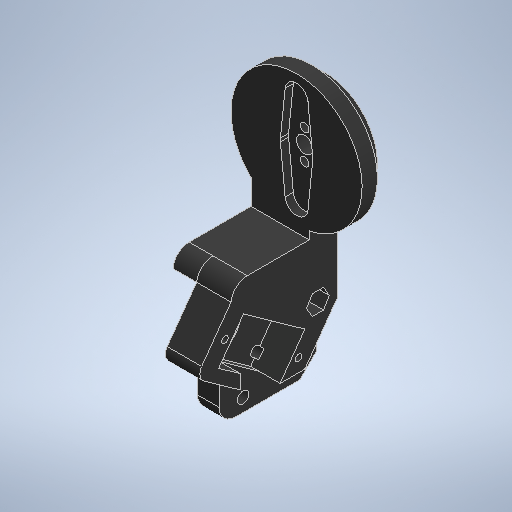
# Autodesk Inventor part: BracoRobotico_0008_001
Saved by Autodesk Inventor 2025.2 (Build 292293000, 293)
## iProperties
Created: 2025-05-22
Part Number: BracoRobotico_0008_001
Material: Rubber
Document SubType Name: Modeling
Designer: I
Density: 0.93 g/cm^3
Appearance: Rubber - Black
Author: I
Autodesk Inventor part; units mm, degrees
sketch "Sketch45" plane through (0, 0, 0) normal (0, 0, 1) x (1, 0, 0)
  circle A0 centre (0, 0) radius 20
  dimension "d321" = 40
  constraints: 1 centre point, 1 coincident
  measures "d321" diameter of A0
extrude "Extrusion48" add sketch "Sketch45" along normal mid plane 8.65
sketch "Sketch49" plane through (0, 0, 4.325) normal (0, 0, 1) x (1, 0, 0)
  circle A0 centre (0, 0) radius 2.5
  circle A1 centre (0, -4.5) radius 1.3
  circle A2 centre (0, 4.5) radius 1.3
  line L0 (0, -4.5) -> (0, 4.5) construction
  circle A3 centre (0, -14) radius 3.5 construction
  circle A4 centre (0, 14) radius 3.5 construction
  line L1 (0, -14) -> (0, 14) construction
  circle A5 centre (0, 0) radius 4.95 construction
  line L2 (-3.4812, -14.3625) -> (-4.9234, -0.5127)
  line L3 (3.4812, -14.3625) -> (4.9234, -0.5127)
  line L4 (-4.9234, 0.5127) -> (-3.4812, 14.3625)
  line L5 (4.9234, 0.5127) -> (3.4812, 14.3625)
  arc A6 (-3.4812, -14.3625) -> (3.4812, -14.3625) centre (0, -14) ccw
  arc A7 (3.4812, 14.3625) -> (-3.4812, 14.3625) centre (0, 14) ccw
  arc A8 (-4.9234, 0.5127) -> (-4.9234, -0.5127) centre (0, 0) ccw
  arc A9 (4.9234, -0.5127) -> (4.9234, 0.5127) centre (0, 0) ccw
  dimension "d338" = 5
  dimension "d339" = 9
  dimension "d340" = 2.6
  dimension "d343" = 7
  dimension "d344" = 28
  dimension "d345" = 9.9
  constraints: 16 point on circle, 12 end point, 10 centre point, 8 tangent, 7 coincident, 2 equal radius, 2 midpoint, 2 vertical
  measures "d338" diameter of A0
  measures "d339" distance of L0.start L0.end
  measures "d340" diameter of A1
  measures "d343" diameter of A4
  measures "d344" distance of L1.start L1.end
  measures "d345" diameter of A5
extrude "Extrusion52" cut sketch "Sketch49" along normal through all both and the other way through all contours A0 | A1 | A2
extrude "Extrusion53" cut sketch "Sketch49" against normal blind 2.5
sketch "Sketch50" plane through (0, 0, -4.325) normal (0, 0, -1) x (-1, 0, 0)
  circle A0 centre (0, -4.5) radius 1.3 construction
  circle A1 centre (0, 4.5) radius 1.3 construction
  circle A2 centre (0, 4.5) radius 3
  circle A3 centre (0, -4.5) radius 3
  point P0 (0, 0)
  dimension "d348" = 6
  constraints: 2 centre point, 2 coincident, 1 equal radius
  measures "d348" diameter of A2
extrude "Extrusion54" cut sketch "Sketch50" against normal blind 3
sketch "Sketch52" plane through (0, 0, -4.325) normal (0, 0, -1) x (-1, 0, 0)
  line L0 (-3.875, -22) -> (13.875, -22)
  line L1 (13.875, -22) -> (13.875, -64)
  line L2 (13.875, -64) -> (-3.875, -64)
  line L3 (-3.875, -64) -> (-3.875, -22)
  line L4 (-3.875, -22) -> (13.875, -64) construction
  line L5 (13.875, -22) -> (-3.875, -64) construction
  point P0 (0, 0)
  point P1 (5, -43)
  dimension "d354" = 17.75
  dimension "d355" = 5
  dimension "d357" = 64
  dimension "d358" = 22
  constraints: 12 end point, 2 midpoint, 1 perpendicular, 1 vertical
  measures "d354" distance of L1.end L2.end
  measures "d355" horizontal distance of point (5, -43) point (0, 0)
  measures "d357" distance from line of point (0, 0) L2
  measures "d358" distance from line of point (0, 0) L0
extrude "Extrusion55" add sketch "Sketch52" against normal blind 40.5
sketch "Sketch54" plane through (0, 0, -4.325) normal (0, 0, -1) x (-1, 0, 0)
  line L0 (13.875, -22) -> (-3.875, -22) projected
  circle A0 centre (0, 0) radius 20 projected
  line L1 (13.875, -22) -> (13.875, -14.4043)
  line L2 (-3.875, -22) -> (-3.875, -19.621)
  constraints: 4 end point, 2 point on circle, 2 vertical
extrude "Extrusion56" add sketch "Sketch54" against normal up to surface (8.65 mm away) contours L0 L2 A0 L1
sketch "Sketch55" plane through (-13.875, -64, -4.325) normal (-1, 0, 0) x (0, 0, 1)
  circle A0 centre (16, 36.748) radius 1.5
  circle A1 centre (16, 11.7287) radius 1.5
  line L0 (0, 0) -> (0, 49.5957) construction
  line L1 (0, 37.5) -> (0, 14.5)
  circle A2 centre (6, 24.2978) radius 1.5
  arc A3 (14.6844, 34.2416) -> (6, 37.5) centre (6, 24.2978) ccw
  line L2 (6, 37.5) -> (0, 37.5)
  line L3 (0, 14.5) -> (1.0053, 13.3867)
  arc A4 (1.0053, 13.3867) -> (14.8889, 16.2363) centre (6, 24.2978) ccw
  arc A5 (17.1111, 16.2363) -> (14.8889, 16.2363) centre (16, 15.2287) ccw
  arc A6 (14.6844, 34.2416) -> (17.3156, 34.2416) centre (16, 35.748) ccw
  circle A7 centre (26, 24.2978) radius 12 construction
  arc A8 (17.1111, 16.2363) -> (29.6085, 12.8532) centre (26, 24.2978) ccw
  arc A9 (26, 37.5) -> (17.3156, 34.2416) centre (26, 24.2978) ccw
  line L4 (26, 37.5) -> (40.5, 37.5)
  line L5 (40.5, 42) -> (40.5, 0) construction
  line L6 (26, 24.2978) -> (29.6085, 12.8532) construction
  line L7 (26, 24.2978) -> (26, 37.5) construction
  line L8 (29.6085, 12.8532) -> (40.5, 12.8532)
  line L9 (40.5, 37.5) -> (40.5, 12.8532)
  point P0 (4.325, 64)
  point P1 (0, 26)
  point P2 (0, 24.7978)
  dimension "d363" = 3
  dimension "d369" = 23
  dimension "d370" = 3
  dimension "d371" = 6
  dimension "d372" = 0.5
  dimension "d375" = 38
  dimension "d377" = 12
  dimension "d378" = 1.5
  dimension "d383" = 1.5
  dimension "d384" = 3.5
  dimension "d385" = 1
  dimension "d386" = 2
  dimension "d388" = 24
  dimension "d389" = 162.5
  dimension "d392" = 20
  constraints: 16 end point, 14 point on circle, 10 centre point, 5 vertical alignment, 4 coincident, 4 point on line, 4 tangent, 3 horizontal, 2 horizontal alignment, 2 midpoint, 1 equal radius
  measures "d363" diameter of A0
  measures "d369" distance of L1.start L1.end
  measures "d370" diameter of A2
  measures "d371" distance from line of L0 A2.centre
  measures "d372" vertical distance of point (0, 24.798) A2.centre
  measures "d375" vertical distance of point (4.325, 64) point (0, 26)
  measures "d377" radius of A4
  measures "d378" distance of L1.end L3.end
  measures "d383" radius of A5
  measures "d384" distance of A1.centre A5.centre
  measures "d385" distance of A0.centre A6.centre
  measures "d386" radius of A6
  measures "d388" diameter of A7
  measures "d389" angle of L7 L6
  measures "d392" distance of A2.centre A7.centre
extrude "Extrusion57" cut sketch "Sketch55" against normal blind 10 contours A0 | A1
extrude "Extrusion58" cut sketch "Sketch55" against normal blind 7.25 contours L2 A3 A6 A9 L4 L9 L8 A8 A5 A4 L3 L1 | A2
extrude "Extrusion59" cut sketch "Sketch55" along normal through all both and the other way through all contours A2
sketch "Sketch56" plane through (-6.625, -22, 4.325) normal (-1, 0, 0) x (0, 0, 1)
  line L0 (32.8095, -17.0077) -> (23.85, -4.5)
  line L1 (23.85, -4.5) -> (23.85, 0)
  line L2 (0, 0) -> (31.85, 0) construction
  line L3 (-8.65, 42) -> (-8.65, 2.379) construction
  line L4 (17.35, -4.5) -> (31.85, -4.5) construction
  arc A0 (32.1118, -21.1977) -> (32.8095, -17.0077) centre (30.3706, -18.7547) ccw
  line L5 (32.1118, -21.1977) -> (20.9585, -29.1468)
  line L6 (20.9585, -29.1468) -> (20.9585, -42)
  line L7 (23.85, 0) -> (35.9585, 0)
  line L8 (35.9585, 0) -> (35.9585, -42)
  line L9 (-8.65, -42) -> (31.85, -42) construction
  line L10 (20.9585, -42) -> (35.9585, -42)
  line L11 (31.85, -4.5) -> (31.85, -29.1468) construction
  line L12 (31.85, -15.6683) -> (31.85, -21.3843)
  point P0 (-4.325, 22)
  point P1 (-8.65, 7.5957)
  point P2 (-8.65, 22.1895)
  point P3 (20.9585, -29.1468)
  point P4 (31.85, -18.5263)
  dimension "d397" = 32.5
  dimension "d398" = 144.385
  dimension "d399" = 3
  dimension "d400" = 125.478
  dimension "d402" = 15
  constraints: 16 end point, 7 point on line, 2 horizontal, 2 midpoint, 2 point on circle, 2 tangent, 1 centre point, 1 coincident, 1 perpendicular, 1 vertical
  measures "d397" distance between parallel lines of L3 L1
  measures "d398" angle of L1 L0
  measures "d399" radius of A0
  measures "d400" angle of L6 L5
  measures "d402" distance of L6.end L8.end
extrude "Extrusion60" cut sketch "Sketch56" along normal through all both and the other way through all contours L0 L1 L7 L8 L10 L6 L5 A0
extrude "Extrusion61" add sketch "Sketch56" against normal up to surface (10.5 mm away) contours A0 L5 L12 L0
sketch "Sketch57" plane through (-13.875, -64, -4.325) normal (-1, 0, 0) x (0, 0, 1)
  circle A0 centre (22.325, 4) radius 1.75
  circle A1 centre (22.325, 4) radius 7 construction
  line L0 (29.6085, 11) -> (26.1971, 9.8315)
  line L1 (29.6085, 0) -> (29.6085, 12.8532) construction
  line L2 (29.6085, 11) -> (29.6085, 0)
  line L3 (22.325, 11) -> (29.6085, 11) construction
  arc A2 (26.1971, 9.8315) -> (15.825, 6.5981) centre (22.325, 4) ccw
  circle A3 centre (9.325, 4) radius 1.75
  arc A4 (15.825, 6.5981) -> (4.3753, 8.9497) centre (9.325, 4) ccw
  arc A5 (1.0053, 13.3867) -> (14.8889, 16.2363) centre (6, 24.2978) ccw construction
  line L4 (9.325, 4) -> (4.3753, 8.9497)
  line L5 (9.325, 4) -> (9.325, 11) construction
  line L6 (4.3753, 8.9497) -> (0, 8.9497)
  line L7 (0, 44.379) -> (0, 0) construction
  line L8 (0, 0) -> (29.6085, 0) projected
  line L9 (0, 8.9497) -> (0, 0)
  line L10 (0, 0) -> (29.6085, 0)
  point P0 (4.325, 64)
  dimension "d407" = 3.5
  dimension "d408" = 14
  dimension "d409" = 60
  dimension "d410" = 18
  dimension "d413" = 18.908
  dimension "d414" = 13
  dimension "d415" = 45
  constraints: 16 end point, 7 point on circle, 5 centre point, 3 coincident, 2 equal radius, 2 horizontal, 2 point on line, 1 horizontal alignment, 1 vertical, 1 vertical alignment
  measures "d407" diameter of A0
  measures "d408" diameter of A1
  measures "d409" vertical distance of point (4.325, 64) A0.centre
  measures "d410" horizontal distance of point (4.325, 64) A0.centre
  measures "d413" angle of L3 L0
  measures "d414" distance of A0.centre A3.centre
  measures "d415" angle of L4 L5
extrude "Extrusion62" cut sketch "Sketch57" against normal blind 4.65
extrude "Extrusion63" cut sketch "Sketch57" against normal through all contours A0 | A3
sketch "Sketch58" plane through (3.875, -64, -4.325) normal (1, 0, 0) x (0, 0, -1)
  circle A0 centre (-6, 24.2978) radius 1.5 construction
  line L0 (-7.7321, 27.2978) -> (-4.2679, 27.2978)
  line L1 (-4.2679, 27.2978) -> (-2.5359, 24.2978)
  line L2 (-2.5359, 24.2978) -> (-4.2679, 21.2978)
  line L3 (-4.2679, 21.2978) -> (-7.7321, 21.2978)
  line L4 (-7.7321, 21.2978) -> (-9.4641, 24.2978)
  line L5 (-9.4641, 24.2978) -> (-7.7321, 27.2978)
  point P0 (-4.325, 64)
  dimension "d420" = 6
  constraints: 12 end point, 1 coincident, 1 horizontal alignment, 13 other
  measures "d420" distance between parallel lines of L2 L5
extrude "Extrusion64" cut sketch "Sketch58" against normal blind 6.5
sketch "Sketch59" plane through (3.875, -64, -4.325) normal (1, 0, 0) x (0, 0, -1)
  line L0 (-36.2611, 21.8926) -> (-28.7161, 32.479)
  line L1 (-28.7161, 32.479) -> (-9.9863, 19.1301)
  line L2 (-9.9863, 19.1301) -> (-17.5313, 8.5437)
  line L3 (-17.5313, 8.5437) -> (-36.2611, 21.8926)
  line L4 (-32.4886, 27.1858) -> (-13.7588, 13.8369) construction
  line L5 (-26.8962, 15.2181) -> (-19.3512, 25.8046) construction
  line L6 (-4.325, -16.8) -> (-4.325, 100.8) construction
  circle A0 centre (-11.8858, 12.502) radius 1
  line L7 (-11.8858, 12.502) -> (-13.7588, 13.8369) construction
  circle A1 centre (-34.3616, 28.5207) radius 1
  line L8 (-32.4886, 27.1858) -> (-34.3616, 28.5207) construction
  line L9 (-40.7618, 20.8023) -> (-29.6085, 12.8532) construction
  line L10 (-32.5, 37.5) -> (-41.4595, 24.9923) construction
  point P0 (-4.325, 64)
  dimension "d423" = 13
  dimension "d424" = 23
  dimension "d427" = 2.3
  dimension "d428" = 2
  dimension "d429" = 3.5
  dimension "d430" = 6
  constraints: 16 end point, 4 midpoint, 3 collinear, 3 perpendicular, 2 centre point, 1 equal radius, 1 parallel
  measures "d423" distance of L0.start L0.end
  measures "d424" distance of L0.end L1.end
  measures "d427" distance of L7.start L4.end
  measures "d428" diameter of A0
  measures "d429" distance between parallel lines of L3 L9
  measures "d430" distance from line of L10 L0.end
extrude "Extrusion65" cut sketch "Sketch59" against normal blind 9 contours L0 L1 L2 L3
extrude "Extrusion66" cut sketch "Sketch59" against normal blind 10 contours A0 | A1
sketch "Sketch60" plane through (-6.625, -64, -4.325) normal (-1, 0, 0) x (0, 0, 1)
  line L0 (36.2611, 21.8926) -> (28.7161, 32.479) projected
  line L1 (28.7161, 32.479) -> (9.9863, 19.1301) projected
  line L2 (17.5313, 8.5437) -> (36.2611, 21.8926) projected
  arc A0 (26, 37.5) -> (17.3156, 34.2416) centre (26, 24.2978) ccw projected
  arc A1 (26, 37.5) -> (17.3156, 34.2416) centre (26, 24.2978) ccw projected
  arc A2 (23.4229, 28.7065) -> (30.9679, 18.1201) centre (27.1954, 23.4133) ccw
  line L3 (36.2611, 21.8926) -> (28.7161, 32.479) projected
  line L4 (32.4886, 27.1858) -> (21.9022, 19.6408) construction
  point P0 (4.325, 64)
  dimension "d437" = 13
  constraints: 3 point on circle, 2 end point, 2 point on line, 2 tangent, 1 centre point, 1 midpoint
  measures "d437" distance of L4.start L4.end
extrude "Extrusion67" cut sketch "Sketch60" against normal through all
sketch "Sketch61" plane through (3.875, -64, -4.325) normal (1, 0, 0) x (0, 0, -1)
  line L0 (-29.6085, 12.8532) -> (-29.6085, 0) projected
  line L1 (0, 0) -> (-29.6085, 0) projected
  line L2 (0, 44.379) -> (0, 0) projected
  line L3 (-9.9863, 19.1301) -> (-17.5313, 8.5437) construction
  line L4 (-17.5313, 8.5437) -> (-36.2611, 21.8926) projected
  line L5 (-29.6085, 12.8532) -> (-29.6085, 17.1512)
  line L6 (-17.5313, 8.5437) -> (-9.9863, 8.5437)
  line L7 (-9.9863, 8.5437) -> (0, 22.5554)
  point P0 (-4.325, 64)
  constraints: 7 end point, 2 point on line, 1 horizontal, 1 parallel, 1 vertical, 1 vertical alignment
extrude "Extrusion68" cut sketch "Sketch61" against normal blind 6.5
chamfer "Chamfer5" distance 1 angle 45 2 edges at (-13.875, -52.2713, 10.175) (-13.875, -27.252, 10.175)
chamfer "Chamfer6" distance 5 angle 45 1 edges at (-5.925, -64, -4.325)
fillet "Fillet12" radius 5 1 edges at (-5.925, -64, 25.2835)
fillet "Fillet13" radius 5 1 edges at (-5, -22, 28.175)
chamfer "Chamfer7" distance 4 angle 45 1 edges at (5.6395, 19.1884, -4.325)
body "Solid4"
